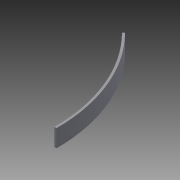
# Autodesk Inventor part: Part13
Saved by Autodesk Inventor 2016 (Build 200138000, 138)
## iProperties
Created: 2016-01-27
Part Number: Part13
Material: Generic
Document SubType Name: Modeling
Designer: 278648
Density: 1 g/cm^3
Appearance: Default
Author: 278648
Autodesk Inventor part; units mm, degrees
ref_plane "YZ Plane" through (0, 0, 0) normal (1, 0, 0) x (0, 1, 0)
ref_plane "XZ Plane" through (0, 0, 0) normal (0, 1, 0) x (-1, 0, 0)
ref_plane "XY Plane" through (0, 0, 0) normal (0, 0, 1) x (1, 0, 0)
sketch "Sketch1" plane through (0, 0, 0) normal (0, 1, 0) x (-1, 0, 0)
  arc A0 (-215.9, 0) -> (-152.6644, -152.6644) centre (0, 0) ccw
  arc A1 (-212.725, 0) -> (-150.4193, -150.4193) centre (0, 0) ccw
  line L0 (-150.4193, -150.4193) -> (-152.6644, -152.6644)
  line L1 (-212.725, 0) -> (-215.9, 0)
  dimension "d0" = 431.8
  dimension "d1" = 3.175
  dimension "d2" = 45
  constraints: 4 end point, 4 point on circle, 2 centre point, 2 coincident, 1 horizontal
  measures "d0" diameter of A0
  measures "d1" radial gap between concentric circles of A0 A1
  measures "d2" angle of L0 L1
extrude "Extrusion1" add sketch "Sketch1" along normal blind 25.4
body "Solid1"
